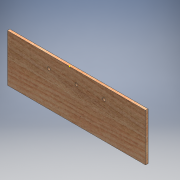
# Autodesk Inventor part: Base
Saved by Autodesk Inventor 2016 (Build 200138000, 138)
## iProperties
Created: 2016-04-01
Part Number: Base
Material: Wood (Birch)
Document SubType Name: Modeling
Designer: mkepler
Density: 0.55 g/cm^3
Appearance: Birch - Natural Polished
Mass: 193.765 g
Surface Area: 997.803 cm^2
Volume: 352.3 cm^3
Author: mkepler
Autodesk Inventor part; units mm, degrees
ref_plane "YZ Plane" through (0, 0, 0) normal (1, 0, 0) x (0, 1, 0)
ref_plane "XZ Plane" through (0, 0, 0) normal (0, 1, 0) x (-1, 0, 0)
ref_plane "XY Plane" through (0, 0, 0) normal (0, 0, 1) x (1, 0, 0)
sketch "Sketch1" plane through (0, 0, 0) normal (0, 1, 0) x (-1, 0, 0)
  line L0 (0, 0) -> (350, 0)
  line L1 (350, 0) -> (350, -120)
  line L2 (350, -120) -> (0, -120)
  line L3 (0, -120) -> (0, 0)
  circle A0 centre (175, -31) radius 3.75
  circle A1 centre (245, -31) radius 3.75
  circle A2 centre (105, -28.4204) radius 3.75
  dimension "d0" = 350
  dimension "d1" = 120
  dimension "d2" = 7.5
  dimension "d3" = 31
  dimension "d4" = 7.5
  dimension "d5" = 7.5
  dimension "d6" = 70
  dimension "d7" = 70
  constraints: 8 end point, 3 centre point, 2 parallel, 1 horizontal, 1 perpendicular
  measures "d0" distance of L1.end L2.end
  measures "d1" distance of L0.end L1.end
  measures "d2" diameter of A0
  measures "d3" distance from line of L0 A0.centre
  measures "d4" diameter of A1
  measures "d5" diameter of A2
  measures "d6" distance of A0.centre A1.centre
  measures "d7" horizontal distance of A0.centre A2.centre
extrude "Extrusion1" add sketch "Sketch1" along normal blind 6.35
sketch "Sketch2" plane through (0, 6.35, 0) normal (0, 1, 0) x (1, 0, 0)
  line L0 (0, 120) -> (-350, 120) projected
  line L1 (-192.5, 120) -> (-157.5, 120)
  line L2 (-157.5, 120) -> (-157.5, 80)
  line L3 (-157.5, 80) -> (-192.5, 80)
  line L4 (-192.5, 80) -> (-192.5, 120)
  line L5 (0, 0) -> (0, 120) projected
  dimension "d10" = 35
  dimension "d11" = 40
  dimension "d12" = 157.5
  constraints: 8 end point, 2 parallel, 1 horizontal, 1 perpendicular, 1 point on line
  measures "d10" distance of L2.end L3.end
  measures "d11" distance of L1.end L2.end
  measures "d12" distance between parallel lines of L5 L2
extrude "Extrusion2" add sketch "Sketch2" along normal blind 62
sketch "Sketch3" plane through (0, 68.35, 0) normal (0, 1, 0) x (1, 0, 0)
  circle A0 centre (-175, 114) radius 2.125
  line L0 (-157.5, 120) -> (-192.5, 120) projected
  circle A1 centre (-169, 114) radius 2.125
  circle A2 centre (-181, 114) radius 2.125
  point P0 (0, 0)
  dimension "d15" = 4.25
  dimension "d16" = 6
  dimension "d17" = 4.25
  dimension "d18" = 6
  dimension "d19" = 4.25
  dimension "d20" = 6
  constraints: 3 centre point
  measures "d15" diameter of A0
  measures "d16" distance from line of L0 A0.centre
  measures "d17" diameter of A1
  measures "d18" distance of A0.centre A1.centre
  measures "d19" diameter of A2
  measures "d20" distance of A0.centre A2.centre
hole "Hole1" at (-181, 68.35, -114) at (-175, 68.35, -114) at (-169, 68.35, -114) direction (0, -1, 0) diameter 4.25 depth 8 tip angle 118
sketch "Sketch4" plane through (-192.5, 6.35, -120) normal (-1, 0, 0) x (0, 0, 1)
  point P0 (120, -6.35)
sketch "Sketch5" plane through (-192.5, 6.35, -120) normal (-1, 0, 0) x (0, 0, 1)
  line L0 (0, 0) -> (0, 62) projected
  line L1 (0, 42) -> (40, 42)
  line L2 (40, 0) -> (40, 62) projected
  line L3 (0, 62) -> (40, 62) projected
  circle A0 centre (6, 48) radius 1.5
  circle A1 centre (34, 48) radius 1.5
  point P0 (120, -6.35)
  dimension "d28" = 20
  dimension "d29" = 3
  dimension "d30" = 3
  dimension "d31" = 6
  dimension "d32" = 6
  dimension "d33" = 6
  dimension "d34" = 6
  constraints: 2 centre point, 2 end point, 2 point on line, 1 horizontal
  measures "d28" distance between parallel lines of L1 L3
  measures "d29" diameter of A0
  measures "d30" diameter of A1
  measures "d31" distance from line of L2 A1.centre
  measures "d32" distance from line of L0 A0.centre
  measures "d33" distance from line of L1 A1.centre
  measures "d34" distance from line of L1 A0.centre
hole "Hole2" at (-192.5, 54.35, -86) at (-192.5, 54.35, -114) direction (1, 0, 0) diameter 3 depth 2 tip angle 118
sketch "Sketch6" plane through (-192.5, 6.35, -80) normal (0, 0, 1) x (1, 0, 0)
  line L0 (0, 42) -> (35, 42)
  line L1 (0, 62) -> (35, 62) projected
  circle A0 centre (6, 48) radius 1.5
  line L2 (0, 0) -> (0, 62) projected
  circle A1 centre (29, 48) radius 1.5
  line L3 (35, 0) -> (35, 62) projected
  point P0 (192.5, -6.35)
  dimension "d42" = 20
  dimension "d43" = 3
  dimension "d44" = 6
  dimension "d45" = 6
  dimension "d46" = 3
  dimension "d47" = 6
  dimension "d48" = 6
  constraints: 2 centre point, 2 end point, 1 horizontal
  measures "d42" distance between parallel lines of L0 L1
  measures "d43" diameter of A0
  measures "d44" distance from line of L2 A0.centre
  measures "d45" distance from line of L0 A0.centre
  measures "d46" diameter of A1
  measures "d47" distance from line of L0 A1.centre
  measures "d48" distance from line of A1.centre L3
hole "Hole3" at (-186.5, 54.35, -80) at (-163.5, 54.35, -80) direction (0, 0, -1) diameter 3 depth 2 tip angle 118
sketch "Sketch7" plane through (-157.5, 6.35, -80) normal (1, 0, 0) x (0, 0, -1)
  circle A0 centre (6, 48) radius 1.5 projected
  circle A1 centre (6, 48) radius 1.5
  circle A2 centre (34, 48) radius 1.5 projected
  circle A3 centre (34, 48) radius 1.5
  point P0 (-80, -6.35)
  dimension "d56" = 3
  dimension "d57" = 3
  constraints: 2 centre point, 2 coincident
  measures "d56" diameter of A1
  measures "d57" diameter of A3
hole "Hole4" at (-157.5, 54.35, -86) at (-157.5, 54.35, -114) direction (-1, 0, 0) diameter 3 depth 2 tip angle 118
body "Solid1"
